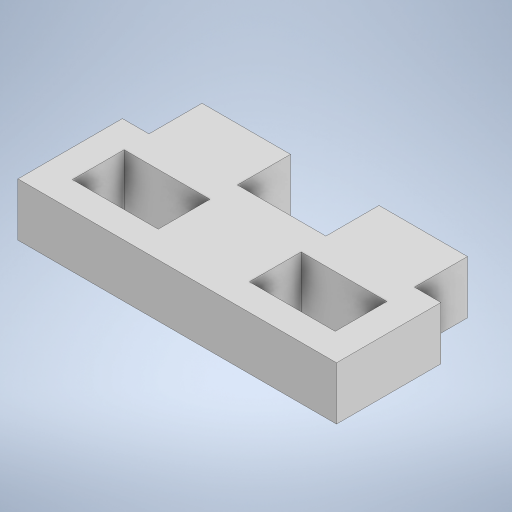
# Autodesk Inventor part: 6mm-Laser-Kerf-Test
Saved by Autodesk Inventor 2023 (Build 270158000, 158)
## iProperties
Created: 2022-11-01
Part Number: 6mm-Laser-Kerf-Test
Material: Generic
Document SubType Name: Modeling
Designer: incep
Density: 1 g/cm^3
Appearance: Default
Author: incep
Autodesk Inventor part; units mm, degrees
ref_plane "YZ Plane" through (0, 0, 0) normal (1, 0, 0) x (0, 1, 0)
ref_plane "XZ Plane" through (0, 0, 0) normal (0, 1, 0) x (-1, 0, 0)
ref_plane "XY Plane" through (0, 0, 0) normal (0, 0, 1) x (1, 0, 0)
sketch "Sketch1" plane through (0, 0, 0) normal (0, 1, 0) x (-1, 0, 0)
  line L0 (-18, -5.8998) -> (-18, 5.8998)
  line L1 (-18, 5.8998) -> (18, 5.8998)
  line L2 (18, 5.8998) -> (18, -5.8998)
  line L3 (15, -11.8998) -> (5, -11.8998)
  line L4 (5, -11.8998) -> (5, -5.8998)
  line L5 (15, -5.8998) -> (15, -11.8998)
  line L6 (18, -5.8998) -> (15, -5.8998)
  line L7 (5, -5.8998) -> (-18, -5.8998) construction
  line L8 (-5, -11.8998) -> (-15, -11.8998)
  line L9 (-15, -11.8998) -> (-15, -5.8998)
  line L10 (-5, -5.8998) -> (-5, -11.8998)
  line L11 (5, -5.8998) -> (-5, -5.8998)
  line L12 (-15, -5.8998) -> (-18, -5.8998)
  line L13 (14.85, -2.9502) -> (5.15, -2.9502)
  line L14 (5.15, -2.9502) -> (5.15, 2.8998)
  line L15 (5.15, 2.8998) -> (14.85, 2.8998)
  line L16 (14.85, 2.8998) -> (14.85, -2.9502)
  line L17 (-5.15, 2.8998) -> (-5.15, -2.9502)
  line L18 (-5.15, -2.9502) -> (-14.85, -2.9502)
  line L19 (-14.85, -2.9502) -> (-14.85, 2.8998)
  line L20 (-14.85, 2.8998) -> (-5.15, 2.8998)
  line L21 (5.15, 2.8998) -> (-5.15, 2.8998) construction
  point P0 (0, 0)
  point P1 (18, 0)
  point P2 (0, -5.8998)
  point P3 (0, 5.8998)
  point P4 (0, 2.8998)
  dimension "d9" = 10
  dimension "d11" = 6
  dimension "d12" = 3
  dimension "d38" = 20
  dimension "d51" = 3
  dimension "d54" = 9.7
  dimension "d55" = 5.85
  dimension "d58" = 20
  dimension "d64" = 3
  constraints: 44 end point, 7 horizontal, 6 parallel, 5 perpendicular, 3 midpoint, 3 vertical alignment, 1 collinear, 1 horizontal alignment, 1 point on line, 15 other
  measures "d9" distance of L3.start L3.end
  measures "d11" distance of L5.start L3.start
  measures "d12" distance between parallel lines of L2 L5
  measures "d38" distance of L3.start L8.start
  measures "d51" distance between parallel lines of L9 L0
  measures "d54" distance of L13.start L13.end
  measures "d55" distance of L15.end L13.start
  measures "d58" distance of L13.start L17.end
  measures "d64" distance between parallel lines of L1 L20
extrude "Extrusion1" add sketch "Sketch1" along normal blind 6
equation "\"d9\" = fingerW"
equation "\"d11\" = fingerH"
equation "\"d38\" = fingerSpacing"
equation "\"d54\" = fingerholeW"
equation "\"d55\" = fingerholeH"
equation "\"d58\" = fingerSpacing"
equation "\"d65\" = thickness"
equation "\"moduleWidth\" = 118"
equation "\"moduleHeight\" = 96"
equation "\"moduleMountD\" = 6.8"
equation "\"moduleCornerR\" = 5"
equation "\"d4\" = moduleCornerR"
equation "\"d5\" = moduleMountD"
equation "\"d6\" = moduleMountD"
equation "\"d8\" = moduleMountD"
equation "\"d10\" = moduleMountD"
equation "\"moduleOpeningR\" = 25"
equation "\"d13\" = moduleOpeningR"
equation "\"thickness\" = 6"
equation "\"d15\" = thickness"
equation "\"d16\" = 0"
equation "\"kerf\" = 0.15"
equation "\"fingerW\" = 10"
equation "\"fingerSpacing\" = 20"
equation "\"fingerholeW\" = fingerW - 2 * kerf"
equation "\"fingerholeH\" = thickness - kerf"
equation "\"moduleMountClearance\" = 19"
equation "\"actuatorW\" = 28"
equation "\"actuatorH\" = 40.8"
equation "\"openingMFC\" = 45"
equation "\"d28\" = thickness"
equation "\"d29\" = thickness"
equation "\"d30\" = 0.5 * actuatorH + thickness"
equation "\"d32\" = fingerholeH"
equation "\"d33\" = fingerholeW"
equation "\"d41\" = fingerholeH"
equation "\"d42\" = fingerholeW"
equation "\"supportSpacingFromMounting\" = 15"
equation "\"d52\" = 58.075"
equation "\"d53\" = 9.475"
equation "\"d0\" = moduleHeight"
equation "\"d1\" = moduleWidth"
equation "\"d17\" = openingMFC"
equation "\"d19\" = moduleMountClearance"
equation "\"d31\" = 15"
equation "\"supportXW\" = -2 * thickness + moduleMountW - 2 * supportSpacingFromMounting + kerf"
equation "\"chairThickness\" = 12.7"
equation "\"supportL\" = -chairThickness + dildoL + actuatorMountL - thickness"
equation "\"fingerH\" = thickness"
equation "\"d18\" = fingerH"
equation "\"d24\" = supportL"
equation "\"d44\" = thickness"
equation "\"d47\" = 0"
equation "\"moduleMountW\" = 100"
equation "\"dildoL\" = 170"
equation "\"actuatorMountL\" = 190"
body "Solid1"
